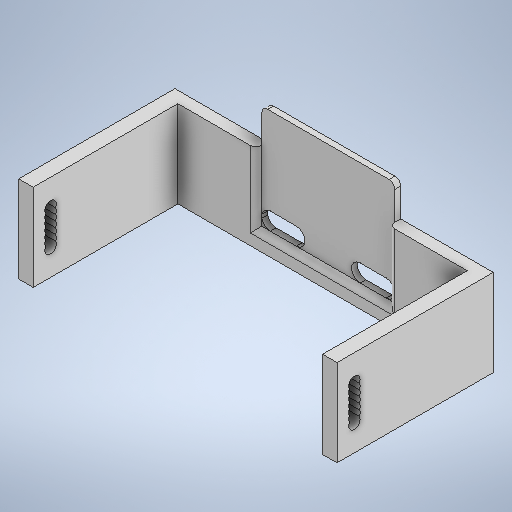
# Autodesk Inventor part: Soporte encoder
Saved by Autodesk Inventor 2025.1 (Build 291241000, 241)
## iProperties
Created: 2025-10-26
Part Number: Soporte encoder
Material: Generic
Document SubType Name: Modeling
Designer: paeze
Density: 1 g/cm^3
Appearance: Default
Author: paeze
Autodesk Inventor part; units mm, degrees
ref_plane "YZ Plane" through (0, 0, 0) normal (1, 0, 0) x (0, 1, 0)
ref_plane "XZ Plane" through (0, 0, 0) normal (0, 1, 0) x (-1, 0, 0)
ref_plane "XY Plane" through (0, 0, 0) normal (0, 0, 1) x (1, 0, 0)
sketch "Sketch1" plane through (0, 0, 0) normal (0, 0, 1) x (1, 0, 0)
  line L0 (-15.8993, 10.1607) -> (7.1007, 10.1607)
  line L1 (7.1007, 10.1607) -> (7.1007, -12.8393)
  line L2 (7.1007, -12.8393) -> (-15.8993, -12.8393)
  line L3 (-15.8993, -12.8393) -> (-15.8993, 10.1607)
  point P0 (0, 0)
  dimension "d0" = 23
  dimension "d1" = 23
  constraints: 8 end point, 2 parallel, 1 horizontal, 1 perpendicular
  measures "d0" distance of L1.end L2.end
  measures "d1" distance of L0.end L1.end
extrude "Extrusion1" add sketch "Sketch1" along normal blind 1
sketch "Sketch2" plane through (0, 0, 1) normal (0, 0, 1) x (1, 0, 0)
  line L0 (-15.8993, -12.8393) -> (7.1007, -12.8393) projected
  line L1 (7.1007, -12.8393) -> (7.1007, 10.1607) projected
  line L2 (-15.8993, -12.8393) -> (7.1007, -12.8393)
  line L3 (7.1007, -12.8393) -> (7.1007, -9.8393)
  line L4 (7.1007, -9.8393) -> (-15.8993, -9.8393)
  line L5 (-15.8993, -9.8393) -> (-15.8993, -12.8393)
  circle A0 centre (-14.4309, -11.3393) radius 1.5
  circle A1 centre (-12.9309, -11.3393) radius 1.5
  circle A2 centre (-11.4309, -11.3393) radius 1.5
  circle A3 centre (-9.9309, -11.3393) radius 1.5
  line L6 (-9.9309, -11.3393) -> (7.1007, -11.3393)
  line L7 (7.1007, -11.3393) -> (4.1007, -11.3393)
  circle A4 centre (5.6007, -11.3393) radius 1.5
  circle A5 centre (4.1007, -11.3393) radius 1.5
  circle A6 centre (2.6007, -11.3393) radius 1.5
  circle A7 centre (1.1007, -11.3393) radius 1.5
  point P0 (0, 0)
  point P1 (-14.4309, -9.8393)
  point P2 (-15.8993, -11.0328)
  point P3 (-15.8993, -11.6457)
  point P4 (-14.4309, -12.8393)
  point P5 (-9.9309, -12.8393)
  point P6 (-9.9309, -9.8393)
  point P7 (5.6007, -9.8393)
  point P8 (1.1007, -9.8393)
  point P9 (1.1007, -12.8393)
  point P10 (5.6007, -12.8393)
  dimension "d5" = 3
  dimension "d6" = 3
  dimension "d11" = 3
  dimension "d12" = 3
  dimension "d4" = 3
  dimension "d7" = 3
  dimension "d8" = 3
  dimension "d9" = 3
  dimension "d10" = 3
  dimension "d13" = 3
  constraints: 12 end point, 4 centre point, 4 point on line, 3 horizontal alignment, 2 midpoint, 2 parallel, 2 point on circle, 1 coincident, 1 horizontal, 1 perpendicular, 9 other
  measures "d4" distance of L3.end L2.end
  measures "d7" diameter of A2
  measures "d8" diameter of A3
  measures "d9" distance of L6.end L7.end
  measures "d10" diameter of A4
  measures "d13" diameter of A7
extrude "Extrusion2" cut sketch "Sketch2" against normal blind 3 contours A0 A1 L0 | A0 L5 A1 | A1 A2 L0 | A1 A0 A2 | A1 A0 | A2 A3 L0 | A2 A1 A3 | A2 A1 | A0 A1 A2 | A0 L4 A1 | A3 A2 L6 | A3 A2 | A1 A2 A3 | A1 L4 A2 | A7 A6 L0 | A7 L6 A6 | L6 A2 A3 | A2 L4 A3 | A6 A5 L0 | A6 A7 A5 | A7 A6 L6 | A6 L6 A7 | A5 A4 L0 | A5 A6 A4 | A5 L6 A6 | A6 A7 L6 | L4 A6 A7 | A5 A6 L6 | A7 A6 A5 | A4 A5 L6 | A4 L6 A5 | A4 A5 L6 | A6 A5 A4 | L4 A5 A6 | L6 A5 A4 | A5 L4 A4
sketch "Sketch3" plane through (0, 0, 0) normal (0, 0, -1) x (-1, 0, 0)
  line L0 (-7.1007, -11.3393) -> (-7.1007, 10.1607) projected
  line L1 (-7.1007, -0.5893) -> (15.8993, -0.5893)
  line L2 (15.8993, -0.5893) -> (15.8993, -12.8393)
  line L3 (15.8993, -12.8393) -> (-7.1007, -12.8393)
  line L4 (-7.1007, -12.8393) -> (-7.1007, -0.5893)
  line L5 (4.3993, -6.7143) -> (4.3993, -12.8393)
  line L6 (4.3993, -6.7143) -> (4.3993, -9.7768)
  line L7 (-13.1007, -0.7455) -> (21.8993, -0.7455)
  line L8 (21.8993, -0.7455) -> (21.8993, -15.7455)
  line L9 (21.8993, -15.7455) -> (-13.1007, -15.7455)
  line L10 (-13.1007, -15.7455) -> (-13.1007, -0.7455)
  line L11 (-13.1007, -0.7455) -> (21.8993, -15.7455) construction
  line L12 (21.8993, -0.7455) -> (-13.1007, -15.7455) construction
  point P0 (0, 0)
  point P1 (4.3993, -8.2455)
  point P2 (15.8993, -0.7455)
  point P3 (-7.1007, -0.7455)
  dimension "d16" = 35
  dimension "d17" = 15
  constraints: 24 end point, 6 midpoint, 4 parallel, 2 horizontal, 2 perpendicular
  measures "d16" distance of L8.end L9.end
  measures "d17" distance of L7.end L8.end
extrude "Extrusion3" add sketch "Sketch3" against normal blind 2 contours L4 L3 L2 L7 L8 L9 L10 L0
sketch "Sketch4" plane through (0, 0, 0) normal (0, 0, -1) x (-1, 0, 0)
  line L0 (-13.1007, -0.7455) -> (-23.1007, -0.7455)
  line L1 (-23.1007, -0.7455) -> (-23.1007, -15.7455)
  line L2 (-23.1007, -15.7455) -> (-13.1007, -15.7455)
  line L3 (-13.1007, -15.7455) -> (-13.1007, -0.7455)
  line L4 (21.8993, -15.7455) -> (21.8993, -0.7455) projected
  line L5 (21.8993, -15.7455) -> (31.8993, -15.7455)
  line L6 (31.8993, -15.7455) -> (31.8993, -0.7455)
  line L7 (31.8993, -0.7455) -> (21.8993, -0.7455)
  line L8 (21.8993, -0.7455) -> (21.8993, -15.7455)
  point P0 (0, 0)
  dimension "d20" = 10
  dimension "d21" = 10
  constraints: 16 end point, 4 parallel, 2 horizontal, 2 perpendicular, 1 point on line
  measures "d20" distance of L2.end L1.end
  measures "d21" distance of L7.end L6.end
extrude "Extrusion4" add sketch "Sketch4" against normal blind 2
sketch "Sketch5" plane through (0, 0, 2) normal (0, 0, 1) x (1, 0, 0)
  line L0 (-31.8993, -0.7455) -> (-31.8993, -15.7455) projected
  line L1 (-31.8993, -15.7455) -> (23.1007, -15.7455) projected
  line L2 (-31.8993, -0.7455) -> (-29.8993, -0.7455)
  line L3 (-29.8993, -0.7455) -> (-29.8993, -15.7455)
  line L4 (-29.8993, -15.7455) -> (-31.8993, -15.7455)
  line L5 (-31.8993, -15.7455) -> (-31.8993, -0.7455)
  line L6 (23.1007, -0.7455) -> (21.1007, -0.7455)
  line L7 (21.1007, -0.7455) -> (21.1007, -15.7455)
  line L8 (21.1007, -15.7455) -> (23.1007, -15.7455)
  line L9 (23.1007, -15.7455) -> (23.1007, -0.7455)
  point P0 (0, 0)
  point P1 (23.1007, -15.7455)
  dimension "d24" = 2
  dimension "d25" = 2
  constraints: 16 end point, 4 parallel, 3 point on line, 2 horizontal, 2 perpendicular
  measures "d24" distance of L3.end L4.end
  measures "d25" distance of L8.end L7.end
extrude "Extrusion5" add sketch "Sketch5" along normal blind 25
sketch "Sketch6" plane through (0, 0, 0) normal (0, 0, -1) x (-1, 0, 0)
  line L0 (-7.1007, -0.7455) -> (-7.1007, 10.1607) projected
  line L1 (15.8993, 10.1607) -> (15.8993, -0.7455) projected
  line L2 (-7.1007, 10.1607) -> (15.8993, 10.1607)
  line L3 (15.8993, 10.1607) -> (15.8993, 5.1607)
  line L4 (15.8993, 5.1607) -> (-7.1007, 5.1607)
  line L5 (-7.1007, 5.1607) -> (-7.1007, 10.1607)
  point P0 (0, 0)
  dimension "d28" = 5
  constraints: 8 end point, 2 parallel, 1 horizontal, 1 perpendicular, 1 point on line
  measures "d28" distance of L2.end L3.end
extrude "Extrusion6" cut sketch "Sketch6" against normal blind 25
fillet "Fillet1" radius 1 5 edges at (7.1007, 5.1607, 0.5) (-15.8993, 5.1607, 0.5) (-15.8993, -6.7924, 2) (7.1007, -6.7924, 2) (-4.3993, -12.8393, 2)
sketch "Sketch7" plane through (0, 0, 27) normal (0, 0, 1) x (1, 0, 0)
  line L0 (6.1007, 5.1607) -> (-14.8993, 5.1607) projected
  line L1 (-4.3993, 5.1607) -> (-4.3993, -15.7455)
  line L2 (-29.8993, -15.7455) -> (21.1007, -15.7455) projected
  line L3 (-4.3993, -5.2924) -> (20.6007, -5.2924)
  line L4 (20.6007, -5.2924) -> (-29.3993, -5.2924)
  line L5 (-16.8993, -0.7455) -> (-29.8993, -0.7455) projected
  line L6 (-29.8993, -0.7455) -> (-29.3993, -0.7455)
  line L7 (-29.3993, -0.7455) -> (-29.3993, -15.7455)
  line L8 (-29.3993, -15.7455) -> (-29.8993, -15.7455)
  line L9 (-29.8993, -15.7455) -> (-29.8993, -0.7455)
  line L10 (21.1007, -0.7455) -> (20.6007, -0.7455)
  line L11 (20.6007, -0.7455) -> (20.6007, -15.7455)
  line L12 (20.6007, -15.7455) -> (21.1007, -15.7455)
  line L13 (21.1007, -15.7455) -> (21.1007, -0.7455)
  point P0 (0, 0)
  dimension "d32" = 25
  dimension "d33" = 50
  constraints: 22 end point, 4 parallel, 4 point on line, 3 horizontal, 3 midpoint, 2 perpendicular
  measures "d32" distance of L3.start L3.end
  measures "d33" distance of L3.end L4.end
extrude "Extrusion7" add sketch "Sketch7" against normal blind 25 contours L11 L10 L13 L2 | L7 L2 L9 L5
sketch "Sketch8" plane through (23.1007, -15.7455, 0) normal (1, 0, 0) x (0, 0, -1)
  line L0 (-27, 15) -> (-27, 0) projected
  line L1 (0, 0) -> (-27, 0) projected
  line L2 (-27, 15) -> (-21, 15)
  line L3 (-21, 15) -> (-21, 0)
  line L4 (-21, 0) -> (-27, 0)
  line L5 (-27, 0) -> (-27, 15)
  line L6 (-24, 15) -> (-24, 0)
  circle A0 centre (-24, 7.5) radius 1
  circle A1 centre (-24, 8.5) radius 1
  circle A2 centre (-24, 9.5) radius 1
  circle A3 centre (-24, 6.5) radius 1
  circle A4 centre (-24, 5.5) radius 1
  circle A5 centre (-24, 4.5) radius 1
  circle A6 centre (-24, 10.5) radius 1
  point P0 (0, 15.7455)
  point P1 (-23.134, 8)
  point P2 (-23.134, 9)
  point P3 (-23.134, 10)
  point P4 (-24.866, 10)
  point P5 (-24.866, 9)
  point P6 (-24.866, 8)
  point P7 (-24.866, 7)
  point P8 (-24.866, 6)
  point P9 (-24.866, 5)
  point P10 (-23.134, 5)
  point P11 (-23.134, 6)
  point P12 (-23.134, 7)
  dimension "d38" = 2
  dimension "d39" = 2
  dimension "d40" = 2
  dimension "d41" = 2
  dimension "d36" = 6
  dimension "d37" = 2
  dimension "d42" = 2
  dimension "d43" = 2
  constraints: 10 end point, 6 point on line, 3 centre point, 3 midpoint, 2 parallel, 2 point on circle, 1 horizontal, 1 perpendicular, 12 other
  measures "d36" distance of L3.end L4.end
  measures "d37" diameter of A0
  measures "d42" diameter of A5
  measures "d43" diameter of A6
extrude "Extrusion8" cut sketch "Sketch8" against normal blind 66.75 contours A6 A2 L6 | L6 A2 A6 | A5 A4 L6 | L6 A4 A5 | A2 A6 L6 | L6 A6 A2 | A6 A1 A2 | A4 A5 L6 | L6 A5 A4 | A4 A3 A5 | A1 A2 L6 | A6 A2 A1 | L6 A2 A1 | A2 A0 A1 | A3 A4 L6 | L6 A4 A3 | A3 A4 A5 | A3 A0 A4 | A0 A1 L6 | A2 A1 A0 | L6 A1 A0 | A1 A3 A0 | A0 A3 L6 | L6 A3 A0 | A0 A3 A4 | A1 A0 A3
equation "\"d14\" = d8"
body "Solid1"
